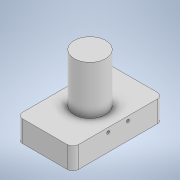
# Autodesk Inventor part: camera_v2
Saved by Autodesk Inventor 2022 (Build 260153000, 153)
## iProperties
Created: 2022-09-26
Part Number: camera_v2
Material: Generic
Document SubType Name: Modeling
Designer: kylem
Density: 1 g/cm^3
Appearance: Default
Author: kylem
Autodesk Inventor part; units mm, degrees
ref_plane "YZ Plane" through (0, 0, 0) normal (1, 0, 0) x (0, 1, 0)
ref_plane "XZ Plane" through (0, 0, 0) normal (0, 1, 0) x (-1, 0, 0)
ref_plane "XY Plane" through (0, 0, 0) normal (0, 0, 1) x (1, 0, 0)
sketch "Sketch1" plane through (0, 0, 0) normal (0, 1, 0) x (-1, 0, 0)
  line L0 (0, 0) -> (58.75, 0)
  line L1 (58.75, 0) -> (58.75, -94.75)
  line L2 (58.75, -94.75) -> (0, -94.75)
  line L3 (0, -94.75) -> (0, 0)
  dimension "d0" = 58.75
  dimension "d1" = 94.75
  constraints: 8 end point, 2 parallel, 1 horizontal, 1 perpendicular
  measures "d0" distance of L1.end L2.end
  measures "d1" distance of L0.end L1.end
extrude "Extrusion1" add sketch "Sketch1" along normal blind 22.6
sketch "Sketch2" plane through (0, 22.6, 0) normal (0, 1, 0) x (1, 0, 0)
  line L0 (-58.75, 0) -> (0, 0) projected
  line L1 (-29.375, 0) -> (-29.375, 94.75)
  line L2 (0, 94.75) -> (-58.75, 94.75) projected
  line L3 (-58.75, 94.75) -> (-58.75, 0) projected
  line L4 (-58.75, 47.375) -> (0, 47.375)
  line L5 (0, 0) -> (0, 94.75) projected
  circle A0 centre (-29.375, 47.375) radius 16.5
  dimension "d4" = 33
  constraints: 5 midpoint, 4 end point, 1 centre point
  measures "d4" diameter of A0
extrude "Extrusion2" add sketch "Sketch2" along normal blind 51 contours A0 L4 L1 | L1 L4 A0 | A0 L1 L4 | L1 A0 L4
fillet "Fillet1" radius 6 4 edges at (0, 11.3, 0) (0, 11.3, -94.75) (-58.75, 11.3, 0) (-58.75, 11.3, -94.75)
sketch "Sketch3" plane through (-58.75, 0, -88.75) normal (-1, 0, 0) x (0, 0, 1)
  line L0 (82.75, 22.6) -> (88.75, 22.6) projected
  line L1 (88.75, 22.6) -> (51.75, 22.6)
  line L2 (24.875, 22.6) -> (57.875, 22.6) projected
  line L3 (51.75, 22.6) -> (51.75, 18.2)
  circle A0 centre (51.75, 18.2) radius 1.5
  line L4 (41.375, 22.6) -> (41.375, 4.2655)
  circle A1 centre (31, 18.2) radius 1.5
  point P0 (88.75, 0)
  dimension "d8" = 37
  dimension "d9" = 4.4
  dimension "d10" = 3
  constraints: 6 end point, 2 centre point, 1 coincident, 1 midpoint, 1 perpendicular, 1 point on line, 1 symmetric about line, 1 vertical, 1 other
  measures "d8" distance of L0.end L1.end
  measures "d9" distance of L1.end L3.end
  measures "d10" diameter of A0
extrude "Extrusion3" cut sketch "Sketch3" against normal blind 70
body "Solid1"
